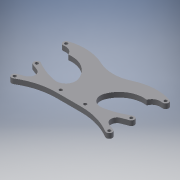
# Autodesk Inventor part: legFrame_Panto
Saved by Autodesk Inventor 2017 (Build 210142000, 142)
## iProperties
Created: 2016-08-27
Part Number: legFrame_Panto
Material: Generic
Document SubType Name: Modeling
Designer: Nic
Density: 1 g/cm^3
Appearance: Default
Author: Nic
Autodesk Inventor part; units mm, degrees
ref_plane "YZ Plane" through (0, 0, 0) normal (1, 0, 0) x (0, 1, 0)
ref_plane "XZ Plane" through (0, 0, 0) normal (0, 1, 0) x (-1, 0, 0)
ref_plane "XY Plane" through (0, 0, 0) normal (0, 0, 1) x (1, 0, 0)
sketch "Sketch1" plane through (0, 0, 0) normal (0, 0, 1) x (1, 0, 0)
  circle A0 centre (0, 0) radius 1.25
  circle A1 centre (-28.6182, 9) radius 1.25
  circle A2 centre (-28.6182, -9) radius 1.25
  line L0 (0, 0) -> (-28.6182, 0) construction
  line L1 (-28.6182, 9) -> (0, 0) construction
  line L2 (-28.6182, 0) -> (-28.6182, 9) construction
  circle A3 centre (0, 0) radius 2.5 construction
  arc A4 (-27.3218, 11.1376) -> (-29.4992, 6.6604) centre (-28.6182, 9) ccw
  arc A5 (-29.4992, -6.6604) -> (-27.3218, -11.1376) centre (-28.6182, -9) ccw
  line L3 (0, 0) -> (0, 7) construction
  line L4 (0, 3.5) -> (10, 3.5) construction
  arc A6 (-27.3218, 11.1376) -> (-12.7131, 5.0568) centre (0, 56.1875) ccw
  line L5 (0, -3.5) -> (10, -3.5)
  line L6 (10, 0) -> (10, 5.5221) construction
  circle A7 centre (20, 0) radius 1.25
  circle A8 centre (48.6182, 9) radius 1.25
  circle A9 centre (48.6182, -9) radius 1.25
  line L7 (20, 0) -> (48.6182, 0) construction
  line L8 (48.6182, 9) -> (20, 0) construction
  line L9 (48.6182, 0) -> (48.6182, 9) construction
  circle A10 centre (20, 0) radius 2.5 construction
  line L10 (20, 0) -> (20, 7) construction
  line L11 (20, 3.5) -> (10, 3.5) construction
  line L12 (20, -3.5) -> (10, -3.5)
  arc A11 (-24.238, -4.6792) -> (-24.238, 4.6792) centre (-26, 0) ccw
  line L13 (-24.238, 4.6792) -> (-29.4992, 6.6604)
  arc A12 (0, -3.5) -> (-27.3218, -11.1376) centre (0, -56.1875) ccw
  line L14 (-24.238, -4.6792) -> (-29.4992, -6.6604)
  arc A13 (32.7131, 5.0568) -> (47.3218, 11.1376) centre (20, 56.1875) ccw
  arc A14 (44.238, 4.6792) -> (44.238, -4.6792) centre (46, 0) ccw
  line L15 (44.238, 4.6792) -> (49.4992, 6.6604)
  arc A15 (47.3218, -11.1376) -> (20, -3.5) centre (20, -56.1875) ccw
  line L16 (44.238, -4.6792) -> (49.4992, -6.6604)
  arc A16 (49.4992, 6.6604) -> (47.3218, 11.1376) centre (48.6182, 9) ccw
  arc A17 (47.3218, -11.1376) -> (49.4992, -6.6604) centre (48.6182, -9) ccw
  circle A18 centre (-36.6182, 37) radius 1.25
  arc A19 (-37.3671, 39.3852) -> (-35.554, 34.7378) centre (-36.6182, 37) ccw
  circle A20 centre (56.6182, 37) radius 1.25
  arc A21 (55.554, 34.7378) -> (57.3671, 39.3852) centre (56.6182, 37) ccw
  arc A22 (-4.0923, 17.2065) -> (-27.067, 28.4144) centre (-25, 3.5) ccw
  arc A23 (47.067, 28.4144) -> (24.0923, 17.2065) centre (45, 3.5) ccw
  arc A24 (-3.7509, 35.3923) -> (12.2087, 31.6729) centre (10, 58.2957) ccw
  arc A25 (12.2087, 31.6729) -> (23.7509, 35.3923) centre (10, 58.2957) ccw
  arc A26 (-12.7131, 5.0568) -> (-4.0923, 17.2065) centre (-10.7828, 12.8204) ccw
  arc A27 (24.0923, 17.2065) -> (32.7131, 5.0568) centre (30.7828, 12.8204) ccw
  arc A28 (-27.067, 28.4144) -> (-35.554, 34.7378) centre (-33, 29.3085) ccw
  arc A29 (55.554, 34.7378) -> (47.067, 28.4144) centre (53, 29.3085) ccw
  arc A30 (-3.7509, 35.3923) -> (-37.3671, 39.3852) centre (-25, 0) ccw
  arc A31 (57.3671, 39.3852) -> (23.7509, 35.3923) centre (45, 0) ccw
  dimension "d0" = 2.5
  dimension "d1" = 9
  dimension "d2" = 30
  dimension "d3" = 5
  dimension "d22" = 3.5
  dimension "d27" = 10
  dimension "d51" = 26
  dimension "d52" = 5
  dimension "d54" = 28
  dimension "d55" = 8
  dimension "d56" = 5
  dimension "d72" = 6
  dimension "d73" = 25
  dimension "d76" = 8
  dimension "d77" = 25
  dimension "d78" = 8
  constraints: 48 point on circle, 34 end point, 32 centre point, 32 symmetric about line, 12 tangent, 9 coincident, 7 equal radius, 3 point on line, 3 vertical, 2 horizontal, 2 vertical alignment, 23 other
  measures "d0" diameter of A0
  measures "d1" distance of L0.end L1.start
  measures "d2" distance of L1.start L0.start
  measures "d3" diameter of A3
  measures "d22" distance from line of point (0, 0) L4
  measures "d27" distance from line of point (0, 0) L6
  measures "d51" distance of point (0, 0) A11.centre
  measures "d52" radius of A11
  measures "d54" vertical distance of L1.start A18.centre
  measures "d55" horizontal distance of A18.centre L1.start
  measures "d56" diameter of A19
  measures "d72" radius of A28
  measures "d73" radius of A22
  measures "d76" horizontal distance of A30.centre A28.centre
  measures "d77" horizontal distance of point (0, 0) A22.centre
  measures "d78" radius of A26
extrude "Extrusion1" add sketch "Sketch1" along normal blind 4
body "Solid1"
